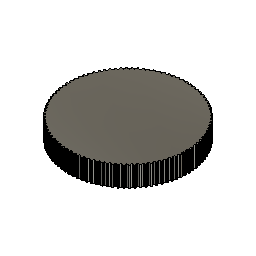
gear_94z (Autodesk Fusion 360 design; units mm, degrees)
Autodesk Fusion 360 part; units mm, degrees
sketch "Sketch1" plane through (0, 0, 0) normal (0, 0, 1) x (1, 0, 0) in component "gt2 pulley"
  circle A0 centre (0, 0) radius 29.9211 construction
  circle A1 centre (0, 0) radius 28.9171 construction
  line L0 (0, 0) -> (0, 29.9211) construction
  line L1 (0, 0) -> (0.9998, 29.9044) construction
  line L2 (0, 0) -> (1.4042, 29.8882) construction
  circle A2 centre (0, 0) radius 29.6671 construction
  arc A3 (0.3976, 29.5315) -> (0.4766, 29.2327) centre (1.3923, 29.6344) ccw
  circle A4 centre (0, 0) radius 29.5171 construction
  arc A5 (0.2496, 29.6661) -> (0, 29.6671) centre (0, 0) ccw
  arc A6 (0.3976, 29.5315) -> (0.2496, 29.6661) centre (0.2484, 29.5161) ccw
  arc A7 (0.4766, 29.2327) -> (0.9663, 28.901) centre (0.9848, 29.4557) ccw
  arc A8 (0, 29.6671) -> (-0.2496, 29.6661) centre (0, 0) ccw
  arc A9 (-0.2496, 29.6661) -> (-0.3976, 29.5315) centre (-0.2484, 29.5161) ccw
  arc A10 (-0.4766, 29.2327) -> (-0.3976, 29.5315) centre (-1.3923, 29.6344) ccw
  arc A11 (-0.9663, 28.901) -> (-0.4766, 29.2327) centre (-0.9848, 29.4557) ccw
  arc A12 (0.9663, 28.901) -> (-0.9663, 28.901) centre (0, 0) ccw
  point P0 (1.3923, 29.6344)
  point P1 (0, 29.6671)
  dimension "d18" = 59.8423
  dimension "d19" = 1.915
  dimension "d22" = 1.004
  dimension "d24" = 0.75
  dimension "d26" = 1
  dimension "d27" = 0.15
  dimension "d28" = 0.15
  dimension "d47" = 0.555
  dimension "d52" = 3.812
  constraint coincident A0.centre A1.centre
  constraint coincident A0 L0.end
  constraint vertical L0
  constraint coincident A0 L1.end
  constraint coincident A0 L2.end
  constraint concentric A1 A2
  constraint coincident A1 A7.end
  constraint coincident L1 A7.end
  constraint coincident A2 P0
  constraint coincident L2 P0
  constraint coincident P0 A3.centre
  constraint coincident A2 P1
  constraint coincident L0 P1
  constraint concentric A2 A4
  constraint coincident P1 A5.end
  constraint coincident A4 A6.centre
  constraint coincident A3.start A6.start
  constraint tangent A3 A6
  constraint tangent A3 A7
  constraint symmetric L0 A7.end A11.start
  constraint symmetric L0 A3.start A9.end
  constraint symmetric L0 A3.end A10.start
  constraint symmetric L0 A3 A10
  constraint symmetric L0 A5.start A8.end
  constraint symmetric L0 P1 A5.end
  constraint symmetric L0 A5 A8
  constraint symmetric L0 A6 A9
  constraint symmetric L0 A7 A11
  constraint coincident A1 A11.start
  constraint tangent A1 A7
  constraint coincident L1 A7.centre
  measures "d18" diameter of A0
  measures "d19" angle of L0 L1
  measures "d22" distance of A0 A1
  measures "d24" distance of A1 A2
  measures "d26" radius of A3
  measures "d27" distance of A2 A4
  measures "d28" radius of A6
  measures "d47" radius of A7
extrude "Extrude1" add sketch "Sketch1" along normal blind 10 makes body 1
pattern_circular "C-Pattern1" count 94 over 360 about axis through (0, 0, 1.75) along (0, 0, 1) of bodies 1 makes body 2 at (-2.6807, 28.7926, 6.6667) makes body 3 at (-3.1081, 28.7496, 3.3333) makes body 4 at (-5.8651, 28.3161, 6.6667) makes body 5 at (-8.3621, 27.6817, 6.6667) makes body 6 at (-9.5869, 27.2817, 6.6667) makes body 7 at (-10.5932, 26.907, 3.3333) makes body 8 at (-13.1377, 25.7605, 6.6667) makes body 9 at (-14.085, 25.255, 3.3333) makes body 10 at (-16.9797, 23.4071, 6.6667) makes body 11 at (-17.3255, 23.1523, 3.3333) makes body 12 at (-18.8332, 21.9434, 3.3333) makes body 13 at (-20.8608, 20.0256, 6.6667) makes body 14 at (-22.1518, 18.5876, 6.6667) makes body 15 at (-22.8266, 17.7523, 3.3333) makes body 16 at (-23.9614, 16.1881, 3.3333) makes body 17 at (-24.9891, 14.5515, 3.3333) makes body 18 at (-26.538, 11.4863, 6.6667) makes body 19 at (-26.7057, 11.0909, 3.3333) makes body 20 at (-27.6504, 8.4648, 6.6667) makes body 21 at (-27.9457, 7.4324, 3.3333) makes body 22 at (-28.532, 4.7038, 6.6667) makes body 23 at (-28.8374, 2.1457, 6.6667) makes body 24 at (-28.9044, 0.8589, 6.6667) makes body 25 at (-28.8972, -1.0736, 6.6667) makes body 26 at (-28.761, -3.0013, 6.6667) makes body 27 at (-28.3797, -5.5493, 6.6667) makes body 28 at (-28.2941, -5.9702, 3.3333) makes body 29 at (-27.8322, -7.8467, 3.3333) makes body 30 at (-26.7057, -11.0909, 6.6667) makes body 31 at (-26.1851, -12.2695, 6.6667) makes body 32 at (-25.3071, -13.9911, 6.6667) makes body 33 at (-24.7702, -14.921, 3.3333) makes body 34 at (-23.2165, -17.2394, 6.6667) makes body 35 at (-22.5604, -18.0894, 6.6667) makes body 36 at (-21.3018, -19.5559, 3.3333) makes body 37 at (-19.3174, -21.5183, 6.6667) makes body 38 at (-17.837, -22.7605, 6.6667) makes body 39 at (-15.7404, -24.2578, 6.6667) makes body 40 at (-14.085, -25.255, 6.6667) makes body 41 at (-12.946, -25.8573, 6.6667) makes body 42 at (-11.19, -26.6643, 6.6667) makes body 43 at (-8.7723, -27.5544, 6.6667) makes body 44 at (-6.9123, -28.0788, 6.6667) makes body 45 at (-5.0214, -28.4778, 6.6667) makes body 46 at (-4.5979, -28.5493, 3.3333) makes body 47 at (-1.8243, -28.8595, 6.6667) makes body 48 at (0.1074, -28.9169, 6.6667) makes body 49 at (2.6807, -28.7926, 6.6667) makes body 50 at (3.1081, -28.7496, 3.3333) makes body 51 at (5.8651, -28.3161, 6.6667) makes body 52 at (8.3621, -27.6817, 6.6667) makes body 53 at (10.1923, -27.0613, 6.6667) makes body 54 at (10.5932, -26.907, 3.3333) makes body 55 at (13.1377, -25.7605, 6.6667) makes body 56 at (14.085, -25.255, 3.3333) makes body 57 at (16.9797, -23.4071, 6.6667) makes body 58 at (17.3255, -23.1523, 3.3333) makes body 59 at (18.8332, -21.9434, 3.3333) makes body 60 at (20.8608, -20.0256, 6.6667) makes body 61 at (21.5899, -19.2374, 3.3333) makes body 62 at (22.8266, -17.7523, 3.3333) makes body 63 at (23.9614, -16.1881, 6.6667) makes body 64 at (25.7115, -13.2332, 6.6667) makes body 65 at (26.538, -11.4863, 6.6667) makes body 66 at (26.7057, -11.0909, 3.3333) makes body 67 at (27.6504, -8.4648, 6.6667) makes body 68 at (28.2941, -5.9702, 6.6667) makes body 69 at (28.532, -4.7038, 6.6667) makes body 70 at (28.7825, -2.7876, 6.6667) makes body 71 at (28.9044, -0.8589, 6.6667) makes body 72 at (28.9163, 0.2148, 3.3333) makes body 73 at (28.8374, 2.1457, 3.3333) makes body 74 at (28.3797, 5.5493, 6.6667) makes body 75 at (28.2941, 5.9702, 3.3333) makes body 76 at (27.8322, 7.8467, 3.3333) makes body 77 at (26.7057, 11.0909, 6.6667) makes body 78 at (26.1851, 12.2695, 6.6667) makes body 79 at (25.3071, 13.9911, 6.6667) makes body 80 at (24.7702, 14.921, 3.3333) makes body 81 at (23.2165, 17.2394, 6.6667) makes body 82 at (22.5604, 18.0894, 3.3333) makes body 83 at (20.2568, 20.6364, 6.6667) makes body 84 at (18.8332, 21.9434, 6.6667) makes body 85 at (17.3255, 23.1523, 6.6667) makes body 86 at (16.2769, 23.9011, 6.6667) makes body 87 at (14.085, 25.255, 6.6667) makes body 88 at (12.3667, 26.1393, 6.6667) makes body 89 at (11.9771, 26.3201, 3.3333) makes body 90 at (10.1923, 27.0613, 3.3333) makes body 91 at (6.9123, 28.0788, 6.6667) makes body 92 at (5.0214, 28.4778, 6.6667) makes body 93 at (3.1081, 28.7496, 6.6667) makes body 94 at (2.6807, 28.7926, 3.3333)
sketch "Sketch2" plane through (0, 0, 10) normal (0, 0, 1) x (-1, 0, 0)
  arc A0 (-10.0627, -27.7671) -> (-9.967, -27.9427) centre (-9.9167, -27.8014) ccw
  arc A1 (-9.967, -27.9427) -> (-9.4954, -28.1065) centre (0, 0) ccw
  arc A2 (-9.4954, -28.1065) -> (-9.3114, -28.0279) centre (-9.4473, -27.9644) ccw
  arc A3 (-9.1389, -27.7716) -> (-9.3114, -28.0279) centre (-8.4055, -28.4515) ccw
  arc A4 (-8.5674, -27.6188) -> (-9.1389, -27.7716) centre (-8.7319, -28.1489) ccw
  arc A5 (-10.393, -26.9849) -> (-8.5674, -27.6188) centre (0, 0) ccw
  arc A6 (-10.0393, -27.4589) -> (-10.393, -26.9849) centre (-10.5925, -27.5028) ccw
  arc A7 (-10.0627, -27.7671) -> (-10.0393, -27.4589) centre (-11.0361, -27.538) ccw
  circle A8 centre (0, 0) radius 28.9171
  constraint coincident A1.centre A5.centre
extrude "Extrude2" add sketch "Sketch2" against normal blind 10 contours A5 A8 bodies 1 2 3 4 5 6 7 8 9 10 11 12 13 14 15 16 17 18 19 20 21 22 23 24 25 26 27 28 29 30 31 32 33 34 35 36 37 38 39 40 41 42 43 44 45 46 47 48 49 50 51 52 53 54 55 56 57 58 59 60 61 62 63 64 65 66 67 68 69 70 71 72 73 74 75 76 77 78 79 80 81 82 83 84 85 86 87 88 89 90 91 92 93 94
extrude "Extrude4" [suppressed] in component "gt2 pulley"
pattern_circular "C-Pattern7" [suppressed] in component "gt2 pulley"
extrude "Extrude3" [suppressed] in component "gt2 pulley"
pattern_circular "C-Pattern6" [suppressed] in component "gt2 pulley"
extrude "Extrude2'" [suppressed] in component "gt2 pulley"
pattern_circular "C-Pattern5" [suppressed] in component "gt2 pulley"
extrude "Extrude1'" [suppressed] in component "gt2 pulley"
pattern_circular "C-Pattern4" [suppressed] in component "gt2 pulley"
pattern_circular "C-Pattern3" [suppressed] in component "gt2 pulley"
pattern_circular "C-Pattern2" [suppressed] in component "gt2 pulley"
pattern_circular "C-Pattern1'" [suppressed] in component "gt2 pulley"
copy_body "Body->Comp1" [suppressed] in component "Component"
copy_body "Body->Comp2" [suppressed] in component "Component'"
copy_body "Body->Comp3" [suppressed] in component "Component''"
copy_body "Body->Comp4" [suppressed] in component "Component'''"
copy_body "Body->Comp5" [suppressed] in component "Component''''"
copy_body "Body->Comp6" [suppressed] in component "Component'''''"
copy_body "Body->Comp7" [suppressed] in component "Component''''''"
copy_body "Body->Comp8" [suppressed] in component "Component'''''''"
copy_body "Body->Comp9" [suppressed] in component "Component''''''''"
copy_body "Body->Comp10" [suppressed] in component "Component'''''''''"
copy_body "Body->Comp11" [suppressed] in component "Component''''''''''"
copy_body "Body->Comp12" [suppressed] in component "Component'''''''''''"
copy_body "Body->Comp13" [suppressed] in component "Component''''''''''''"
copy_body "Body->Comp14" [suppressed] in component "Component'''''''''''''"
copy_body "Body->Comp15" [suppressed] in component "Component''''''''''''''"
copy_body "Body->Comp16" [suppressed] in component "Component'''''''''''''''"
copy_body "Body->Comp17" [suppressed] in component "Component''''''''''''''''"
copy_body "Body->Comp18" [suppressed] in component "Component'''''''''''''''''"
copy_body "Body->Comp19" [suppressed] in component "Component''''''''''''''''''"
copy_body "Body->Comp20" [suppressed] in component "Component'''''''''''''''''''"
component "gt2 pulley" placed x (1, 0, 0) y (0, 1, 0) z (0, 0, 1) at (0, 0, 0)
equation "NumTeeth = 94" comment "min 20"
equation "ToothPitch = 2 mm"
equation "PullyDia = NumTeeth * ToothPitch / PI"
equation "ToothAng = ( ( 360 / NumTeeth ) * 1 deg )"
equation "TransOffsetAngle = ToothAng * 0.2"
equation "Sholulder_Radius = 0.15 mm"
equation "Root_Radius = 0.555 mm"
equation "TransRadius = 1 mm"
equation "ToolHeight = 0.75 mm"
equation "PLD = 0.254 mm"
equation "d18 = PullyDia"
equation "d19 = ToothAng / 2"
equation "d22 = PLD + ToolHeight"
equation "d24 = ToolHeight"
equation "d26 = TransRadius"
equation "d27 = Sholulder_Radius"
equation "d31 = NumTeeth"
equation "d33 = NumTeeth"
equation "d35 = NumTeeth"
equation "d37 = NumTeeth"
equation "d41 = NumTeeth"
equation "d45 = NumTeeth"
equation "d47 = Root_Radius"
equation "d50 = NumTeeth"
